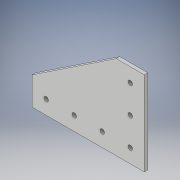
# Autodesk Inventor part: Drivetrain_gussets
Saved by Autodesk Inventor 2018 (Build 220112000, 112)
## iProperties
Created: 2018-09-06
Part Number: Drivetrain_gussets
Material: Generic
Document SubType Name: Modeling
Designer: baoan
Density: 1 g/cm^3
Appearance: Default
Author: baoan
Autodesk Inventor part; units mm, degrees
ref_plane "YZ Plane" through (0, 0, 0) normal (1, 0, 0) x (0, 1, 0)
ref_plane "XZ Plane" through (0, 0, 0) normal (0, 1, 0) x (-1, 0, 0)
ref_plane "XY Plane" through (0, 0, 0) normal (0, 0, 1) x (1, 0, 0)
sketch "Sketch1" plane through (0, 0, 0) normal (0, 0, 1) x (1, 0, 0)
  line L0 (-50.8, -38.1) -> (50.8, -38.1)
  line L1 (50.8, -38.1) -> (50.8, 38.1)
  line L2 (50.8, 38.1) -> (25.4, 38.1)
  line L3 (-50.8, 38.1) -> (-50.8, -12.7) construction
  line L4 (-50.8, -38.1) -> (50.8, 38.1) construction
  line L5 (50.8, -38.1) -> (-50.8, 38.1) construction
  line L6 (-50.8, -12.7) -> (25.4, 38.1)
  line L7 (25.4, 38.1) -> (-50.8, 38.1) construction
  line L8 (-50.8, -12.7) -> (-50.8, -38.1)
  point P0 (0, 0)
  dimension "d0" = 101.6
  dimension "d1" = 76.2
  dimension "d2" = 25.4
  dimension "d3" = 25.4
  constraints: 18 end point, 4 parallel, 2 midpoint, 1 horizontal, 1 perpendicular
  measures "d0" distance of L3.start L1.end
  measures "d1" distance of L1.end L0.end
  measures "d2" distance of L1.end L2.end
  measures "d3" distance of L0.start L3.end
extrude "Extrusion1" add sketch "Sketch1" along normal mid plane 3.175
sketch "Sketch2" plane through (0, 0, 1.5875) normal (0, 0, 1) x (1, 0, 0)
  line L0 (50.8, -38.1) -> (50.8, 38.1) projected
  line L1 (50.8, 38.1) -> (25.4, 38.1) projected
  point P0 (0, 0)
  point P1 (38.1, 25.4)
  point P2 (38.1, 0)
  point P3 (38.1, -25.4)
  point P4 (12.7, -25.4)
  point P5 (-12.7, -25.4)
  point P6 (-38.1, -25.4)
  dimension "d6" = 25.4
  dimension "d7" = 25.4
  dimension "d8" = 25.4
  dimension "d9" = 12.7
  dimension "d10" = 25.4
  dimension "d11" = 25.4
  dimension "d12" = 12.7
  constraints: 3 horizontal alignment, 2 vertical alignment
  measures "d6" distance of point (-12.7, -25.4) point (-38.1, -25.4)
  measures "d7" distance of point (12.7, -25.4) point (-12.7, -25.4)
  measures "d8" distance of point (38.1, -25.4) point (12.7, -25.4)
  measures "d9" distance from line of L0 point (38.1, -25.4)
  measures "d10" distance of point (38.1, -25.4) point (38.1, 0)
  measures "d11" distance of point (38.1, 25.4) point (38.1, 0)
  measures "d12" distance from line of L1 point (38.1, 25.4)
hole "Hole1" at (38.1, 25.4, 1.5875) at (38.1, 0, 1.5875) at (38.1, -25.4, 1.5875) at (12.7, -25.4, 1.5875) at (-12.7, -25.4, 1.5875) at (-38.1, -25.4, 1.5875) direction (0, 0, -1) diameter 4.1402 end through all
body "Solid1"
